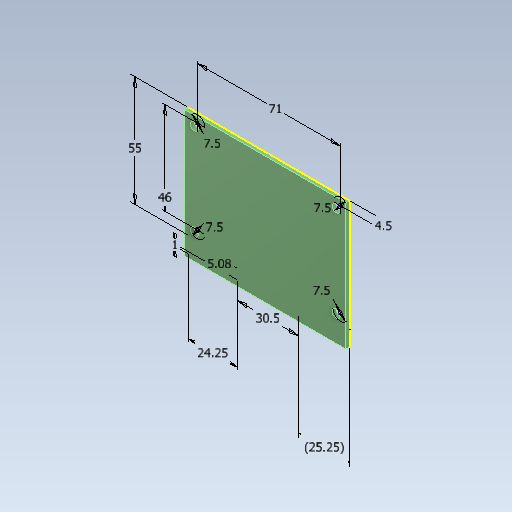
# Autodesk Inventor part: Sensor Head PCB
Saved by Autodesk Inventor 2021 (Build 250183000, 183)
## iProperties
Created: 2019-11-04
Part Number: Sensor Head PCB
Material: Generic
Document SubType Name: Modeling
Designer: jgray
Density: 1 g/cm^3
Appearance: White
Author: jgray
Autodesk Inventor part; units mm, degrees
ref_plane "YZ Plane" through (0, 0, 0) normal (1, 0, 0) x (0, 1, 0)
ref_plane "XZ Plane" through (0, 0, 0) normal (0, 1, 0) x (-1, 0, 0)
ref_plane "XY Plane" through (0, 0, 0) normal (0, 0, 1) x (1, 0, 0)
sketch "Sketch1" plane through (0, 0, 0) normal (0, 0, 1) x (1, 0, 0)
  line L0 (0, 0) -> (80, 0)
  line L1 (80, 0) -> (80, 63)
  line L2 (80, 63) -> (0, 63)
  line L3 (0, 63) -> (0, 0)
  line L4 (4.75, 58.25) -> (75.25, 58.25) construction
  line L5 (75.25, 58.25) -> (75.25, 12.75) construction
  line L6 (75.25, 12.75) -> (4.75, 12.75) construction
  line L7 (4.75, 12.75) -> (4.75, 58.25) construction
  dimension "d0" = 80
  dimension "d1" = 63
  dimension "d2" = 70.5
  dimension "d3" = 45.5
  dimension "d4" = 4.75
  dimension "d5" = 4.75
  dimension "d6" = 4.75
  constraints: 16 end point, 4 coincident, 4 parallel, 2 horizontal, 2 perpendicular
  measures "d0" distance of L2.end L1.end
  measures "d1" distance of L1.end L0.end
  measures "d2" distance of L5.end L6.end
  measures "d3" distance of L4.end L5.end
  measures "d4" distance between parallel lines of L3 L7
  measures "d5" distance between parallel lines of L1 L5
  measures "d6" distance between parallel lines of L2 L4
extrude "Extrusion1" add sketch "Sketch1" along normal blind 1.8
hole "Hole1" at (75.25, 58.25, 0) at (4.75, 58.25, 0) at (4.75, 12.75, 0) at (75.25, 12.75, 0) direction (0, 0, 1) diameter 4 end through all
sketch "Sketch2" plane through (0, 0, 0) normal (0, 0, -1) x (-1, 0, 0)
  line L0 (-54.75, 6.08) -> (-24.25, 6.08)
  line L1 (-24.25, 6.08) -> (-24.25, 1)
  line L2 (-24.25, 1) -> (-54.75, 1)
  line L3 (-54.75, 1) -> (-54.75, 6.08)
  line L4 (0, 0) -> (-80, 0) projected
  line L5 (0, 63) -> (0, 0) projected
  line L6 (-80, 0) -> (-80, 63) projected
  line L7 (-80, 0) -> (-80, 63) projected
  line L8 (-80, 8) -> (0, 8)
  line L9 (0, 63) -> (0, 0) projected
  line L10 (-80, 63) -> (0, 63) projected
  line L11 (-71.75, 58.5) -> (-8.25, 58.5)
  line L12 (-4.5, 54.75) -> (-4.5, 16.25)
  line L13 (-8.25, 12.5) -> (-71.75, 12.5)
  line L14 (-75.5, 16.25) -> (-75.5, 54.75)
  line L15 (0, 0) -> (-80, 0) construction
  line L16 (-40, 0) -> (-40, 63) construction
  arc A0 (-8.25, 58.5) -> (-4.5, 54.75) centre (-4.5, 58.5) ccw
  arc A1 (-75.5, 54.75) -> (-71.75, 58.5) centre (-75.5, 58.5) ccw
  arc A2 (-71.75, 12.5) -> (-75.5, 16.25) centre (-75.5, 12.5) ccw
  arc A3 (-4.5, 16.25) -> (-8.25, 12.5) centre (-4.5, 12.5) ccw
  dimension "d16" = 30.5
  dimension "d17" = 5.08
  dimension "d18" = 1
  dimension "d19" = 24.25
  dimension "d20" = 25.25
  dimension "d21" = 55
  dimension "d24" = 4.5
  dimension "d25" = 7.5
  dimension "d26" = 7.5
  dimension "d27" = 7.5
  dimension "d28" = 7.5
  dimension "d29" = 71
  dimension "d30" = 46
  constraints: 20 end point, 8 point on circle, 4 centre point, 4 parallel, 3 perpendicular, 2 horizontal, 2 midpoint, 2 point on line, 1 other
  measures "d16" distance of L1.end L2.end
  measures "d17" distance of L0.end L1.end
  measures "d18" distance between parallel lines of L4 L2
  measures "d19" distance between parallel lines of L5 L1
  measures "d20" distance between parallel lines of L3 L6
  measures "d21" distance between parallel lines of L8 L10
  measures "d24" distance between parallel lines of L10 L11
  measures "d25" diameter of A0
  measures "d26" diameter of A1
  measures "d27" diameter of A2
  measures "d28" diameter of A3
  measures "d29" distance between parallel lines of L12 L14
  measures "d30" distance between parallel lines of L13 L11
body "Solid1"
